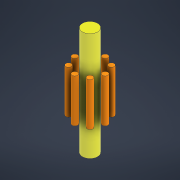
# Autodesk Inventor part: 110033226_ipt_53_散步橋圓柱
Saved by Autodesk Inventor 2022 (Build 260153000, 153)
## iProperties
Created: 2022-06-30
Part Number: 110033226_ipt_53_散步橋圓柱
Material: 一般
Document SubType Name: Modeling
Designer: User
Density: 1 g/cm^3
Appearance: 預設
Author: User
Autodesk Inventor part; units mm, degrees
ref_plane "YZ Plane" through (0, 0, 0) normal (1, 0, 0) x (0, 1, 0)
ref_plane "XZ Plane" through (0, 0, 0) normal (0, 1, 0) x (-1, 0, 0)
ref_plane "XY Plane" through (0, 0, 0) normal (0, 0, 1) x (1, 0, 0)
sketch "草圖1" plane through (0, 0, 0) normal (0, 1, 0) x (-1, 0, 0)
  circle A0 centre (0, 0) radius 1.75
  dimension "d0" = 3.5
  constraints: 1 centre point, 1 coincident
  measures "d0" diameter of A0
extrude "擠出1" add sketch "草圖1" along normal blind 25
ref_plane "工作平面1" through (0, 12.5, 0) normal (0, 1, 0) x (1, 0, 0)
sketch "草圖2" plane through (0, 12.5, 0) normal (0, 1, 0) x (1, 0, 0)
  circle A0 centre (0, 0) radius 1.75 projected
  circle A1 centre (0, 0) radius 3.5
  circle A2 centre (3.5, 0) radius 0.65
  dimension "d3" = 7
  dimension "d4" = 1.3
  constraints: 1 centre point, 1 coincident, 1 horizontal alignment, 2 other
  measures "d4" diameter of A2
extrude "擠出2" add sketch "草圖2" along normal mid plane 10 contours A1 A2 | A1 A2 picked at (3.2876, -0.1251) picked at (3.6904, -0.1714)
pattern_circular "環形陣列1" count 8 over 360 about axis through (0, 0, 0) along (0, 1, 0) of "擠出2"
